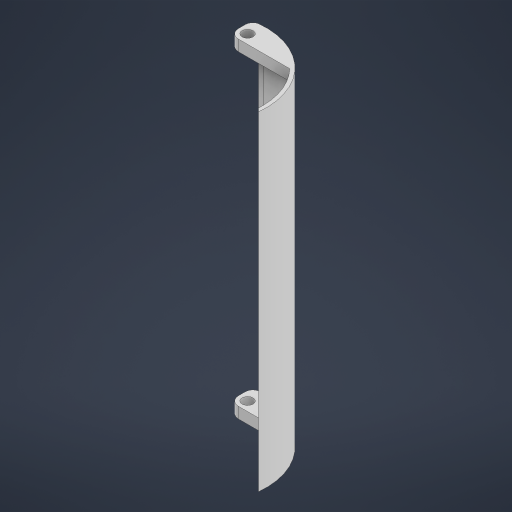
# Autodesk Inventor part: wind blade
Saved by Autodesk Inventor 2024 (Build 280153000, 153)
## iProperties
Created: 2023-07-13
Part Number: wind blade
Material: 일반
Document SubType Name: Modeling
Designer: 6gioc
Density: 1 g/cm^3
Appearance: 기본값
Author: 6gioc
Autodesk Inventor part; units mm, degrees
ref_plane "YZ Plane" through (0, 0, 0) normal (1, 0, 0) x (0, 1, 0)
ref_plane "XZ Plane" through (0, 0, 0) normal (0, 1, 0) x (-1, 0, 0)
ref_plane "XY Plane" through (0, 0, 0) normal (0, 0, 1) x (1, 0, 0)
sketch "스케치1" plane through (0, 0, 0) normal (0, 1, 0) x (-1, 0, 0)
  arc A0 (0, 0) -> (17.6777, -17.6777) centre (17.9972, 0.3195) ccw
  line L0 (0, 0) -> (17.6777, -17.6777) construction
  line L1 (0, 0) -> (25, 0) construction
  arc A1 (-0.898, 2.3123) -> (19.9899, -18.5757) centre (17.9972, 0.3195) ccw
  line L2 (-0.898, 2.3123) -> (19.9899, -18.5757)
  line L3 (0, 0) -> (0, 1.4142)
  line L4 (17.6777, -17.6777) -> (19.0919, -17.6777)
  dimension "d0" = 25
  dimension "d1" = 45
  dimension "d2" = 18
  dimension "d3" = 1
  constraints: 10 end point, 4 point on circle, 2 centre point, 2 point on line, 1 equal length, 1 horizontal, 1 perpendicular, 1 vertical, 1 other
  measures "d0" distance of L0.start L0.end
  measures "d1" angle of L0 L1
  measures "d2" radius of A0
  measures "d3" radial gap between concentric circles of A0 A1
extrude "돌출1" add sketch "스케치1" along normal blind 90 contours A0 L4 L2 A1 L3
sketch "스케치2" plane through (0, 0, 0) normal (0, -1, 0) x (1, 0, 0)
  circle A0 centre (-19.0919, -14.6777) radius 1.5
  arc A1 (-17.6777, -17.6777) -> (0, 0) centre (-17.9972, 0.3195) ccw projected
  circle A2 centre (-19.0919, -14.6777) radius 2.5
  line L0 (-19.0919, -12.1777) -> (-5.0426, -12.1777)
  line L1 (-21.5919, -14.6777) -> (-21.5919, -18.2148)
  line L2 (-21.5919, -14.6777) -> (-18.0548, -14.6777) construction
  line L3 (-19.9899, -18.5757) -> (-19.0919, -17.6777) projected
  line L4 (-19.9899, -18.5757) -> (-21.5919, -18.5757)
  line L5 (-21.5919, -18.5757) -> (-21.5919, -18.2148)
  line L6 (0, 0) -> (0, 1.4142) projected
  line L7 (0, 1.4142) -> (0.898, 2.3123) projected
  arc A3 (-19.9899, -18.5757) -> (0.898, 2.3123) centre (-17.9972, 0.3195) ccw projected
  line L8 (-19.9899, -18.5757) -> (-19.0919, -17.6777) projected
  line L9 (-19.0919, -17.6777) -> (-17.6777, -17.6777) projected
  arc A4 (-17.6777, -17.6777) -> (0, 0) centre (-17.9972, 0.3195) ccw projected
  point P0 (-17.6777, -17.6777)
  dimension "d6" = 3
  dimension "d7" = 3
  dimension "d8" = 1
  dimension "d9" = 90
  constraints: 10 end point, 3 horizontal, 3 point on circle, 2 centre point, 2 perpendicular, 2 tangent, 1 vertical alignment
  measures "d6" diameter of A0
  measures "d7" distance of L3.end A0.centre
  measures "d8" radial gap between concentric circles of A0 A2
  measures "d9" angle of L1 L2
extrude "돌출2" add sketch "스케치2" against normal blind 3 contours L9 L3 L4 L5 L1 A2 L0 A1 | A2
fillet "모깎기1" radius 2 1 edges at (-21.5919, 1.5, -18.5757)
sketch "스케치3" plane through (0, 90, 0) normal (0, 1, 0) x (1, 0, 0)
  arc A0 (-19.9899, 18.5757) -> (-21.5919, 16.6157) centre (-19.5919, 16.6157) ccw projected
  line L0 (-21.5919, 16.6157) -> (-21.5919, 14.6777) projected
  arc A1 (-21.5919, 14.6777) -> (-19.0919, 12.1777) centre (-19.0919, 14.6777) ccw projected
  line L1 (-19.0919, 12.1777) -> (-5.0426, 12.1777) projected
  arc A2 (-5.0426, 12.1777) -> (-17.6777, 17.6777) centre (-17.9972, -0.3195) ccw projected
  line L2 (-19.0919, 17.6777) -> (-17.6777, 17.6777) projected
  line L3 (-19.9899, 18.5757) -> (-19.0919, 17.6777) projected
  circle A3 centre (-19.0919, 14.6777) radius 1.5 projected
  point P0 (0, 0)
extrude "돌출3" add sketch "스케치3" against normal blind 3
